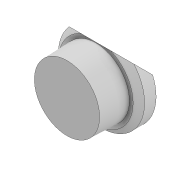
# Autodesk Inventor part: tmp_20_Cube_Insert_Kinematic_Astromedia_30x40x90_pro_magnetic_M12lens_mirrormount
Saved by Autodesk Inventor 2022 (Build 260153000, 153)
## iProperties
Created: 2023-01-01
Part Number: tmp_20_Cube_Insert_Kinematic_Astromedia_30x40x90_pro_magnetic_M12lens_mirrormount
Material: Generisch
Document SubType Name: Modeling
Designer: diederichbenedict
Density: 1 g/cm^3
Appearance: Vorgabe
Author: diederichbenedict
Autodesk Inventor part; units mm, degrees
ref_plane "YZ Plane" through (0, 0, 0) normal (1, 0, 0) x (0, 1, 0)
ref_plane "XZ Plane" through (0, 0, 0) normal (0, 1, 0) x (-1, 0, 0)
sketch "Skizze1" plane through (0, 0, 0) normal (0, 1, 0) x (-1, 0, 0)
  point P0 (0, 0)
sketch "Skizze2" plane through (0, 0, 0) normal (0, 0, 1) x (1, 0, 0)
  circle A0 centre (0, 0) radius 5.85
  dimension "d0" = 11.7
  constraints: 1 centre point, 1 coincident
  measures "d0" diameter of A0
extrude "Extrusion1" add sketch "Skizze2" along normal blind 5 draft -2
sketch "Skizze3" plane through (0, 0, 0) normal (0, 0, -1) x (-1, 0, 0)
  circle A0 centre (0, 0) radius 7.5
  dimension "d3" = 15
  constraints: 1 centre point, 1 coincident
  measures "d3" diameter of A0
extrude "Extrusion2" add sketch "Skizze3" along normal blind 1
sketch "Skizze4" plane through (0, 0, -1) normal (0, 0, -1) x (-1, 0, 0)
  circle A0 centre (0, 0) radius 7.5 projected
ref_plane "Arbeitsebene1" through (-5, -7, -5.9) normal (0, 0, 1) x (1, 0, 0)
extrude "Extrusion3" add sketch "Skizze4" along normal blind 4
chamfer "Fase1" distance 1 angle 45 1 edges at (7.5, 0, 0)
sketch "Skizze5" plane through (0, 0, 0) normal (1, 0, 0) x (0, 1, 0)
  line L0 (-7.5, -1) -> (-7.5, -5) projected
  line L1 (-7.5, -3) -> (2.9599, -3)
  line L2 (2.9599, -3) -> (7.8543, 1.8945)
  line L3 (7.8543, 1.8945) -> (7.8543, -11.1641)
  line L4 (7.8543, -11.1641) -> (-9.215, -10.2828)
  line L5 (-9.215, -10.2828) -> (-7.5, -3)
  point P0 (0, 0)
  dimension "d11" = 135
  constraints: 10 end point, 1 horizontal, 1 midpoint, 1 perpendicular
  measures "d11" angle of L2 L1
extrude "Extrusion4" cut sketch "Skizze5" along normal through all both and the other way through all
